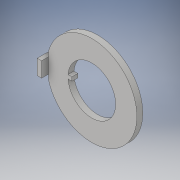
# Autodesk Inventor part: AT507H
Saved by Autodesk Inventor 2019 (Build 230136000, 136)
## iProperties
Created: 2022-08-22
Part Number: AT507H
Material: Generic
Catalog Web Link: www.cadenas.de
Description: Locking Ring - Bushing Mount Miniature Toggles-Series M - Standard Hardwarw for Small & Large Bushings
Vendor: NKKSWITCHES
Document SubType Name: Modeling
Designer: psAdmin
Manufacturer: NKKSWITCHES
Mass: 0.0656955 g
Surface Area: 2.15721 cm^2
Volume: 0.0656955 cm^3
Density: 1 g/cm^3
Appearance: PSOLRGB-175-175-175
Category: PARTsolutions
Company: NKKSWITCHES
Title: AT507H
Author: Cadenas PARTsolutions
Comments: Series M - Standard Hardwarw for Small & Large Bushings
PSOL_IDENT_0: {$CADENAS_DATA/23d-libs/nkkswitches/toggle/m/hardware/locking_ring.prj},192 {VTYP=3D},{NB=AT507H},{L
PSOL_IDENT_1: INA=AT507H},{NN=Locking Ring - Bushing Mount Miniature Toggles},{DATE=02.08.2022 07:27:09},{GEOMDATE=
PSOL_IDENT_2: 12.04.2007 13:28:00},{VERSION=},{LINEID=10},{WBVAR=},{WBNUMERIC=}  {NB=AT507H},{LINA=AT507H},{KT=DUM
PSOL_IDENT_3: MY},{PN=AT507H},{A=0.079},{B=0.229},{D=0.472},{DD=0.250},{T=0.031},{TT=0.067},{T1=0.023},{LC=0.486},
PSOL_IDENT_4: {T2=0.020}
NB: AT507H
NN: Locking Ring - Bushing Mount Miniature Toggles
NT: Series M - Standard Hardwarw for Small & Large Bushings
NBSYN: $PN.
LINA: AT507H
CATALOG: NKK Switches
PN: AT507H
T1: 0.023
LC: 0.486
T2: 0.02
SUPPLIER: NKKSWITCHES
ARTICLENO: AT507H
BOMINFO: AT507H
CREATOR: CADENAS GmbH
Autodesk Inventor part; units mm, degrees
sketch "Sketch_4" plane through (0, 0, 0) normal (0, 0, 1) x (1, 0, 0)
  line L0 (-5.7658, 1.6396) -> (-5.7658, -1.6396)
  arc A0 (-5.7658, -1.6396) -> (-5.7658, 1.6396) centre (0, 0) ccw
  arc A1 (-3.1648, -0.254) -> (-3.1648, 0.254) centre (0, 0) ccw
  line L1 (-3.1648, 0.254) -> (-2.6416, 0.254)
  line L2 (-2.6416, 0.254) -> (-2.6416, -0.254)
  line L3 (-2.6416, -0.254) -> (-3.1648, -0.254)
  constraints: 8 end point, 4 point on circle, 2 centre point
extrude "Extrusion1" add sketch "Sketch_4" along normal blind 0.7874
sketch "Sketch_2" plane through (0, 0, 0) normal (0, 1, 0) x (-1, 0, 0)
  line L0 (6.35, 0.3937) -> (6.35, 1.7018)
  line L1 (6.35, 1.7018) -> (5.7658, 1.7018)
  line L2 (5.7658, 1.7018) -> (5.7658, 0.7874)
  line L3 (5.7658, 0.7874) -> (4.4069, 0.7874)
  line L4 (4.4069, 0.7874) -> (4.4069, 0)
  line L5 (4.4069, 0) -> (5.9563, 0)
  arc A0 (5.9563, 0) -> (6.35, 0.3937) centre (5.9563, 0.3937) ccw
  constraints: 12 end point, 2 point on circle, 1 centre point
extrude "Extrusion2" add sketch "Sketch_2" along normal mid plane 2.0066
ref_plane "ring_XY" through (0, 0, 0.3937) normal (0, 0, 1) x (1, 0, 0)
ref_plane "ring_YZ" through (0, 0, 0.3937) normal (1, 0, 0) x (0, 1, 0)
ref_plane "ring_ZX" through (0, 0, 0.3937) normal (0, 1, 0) x (0, 0, 1)
body "Solid1"
